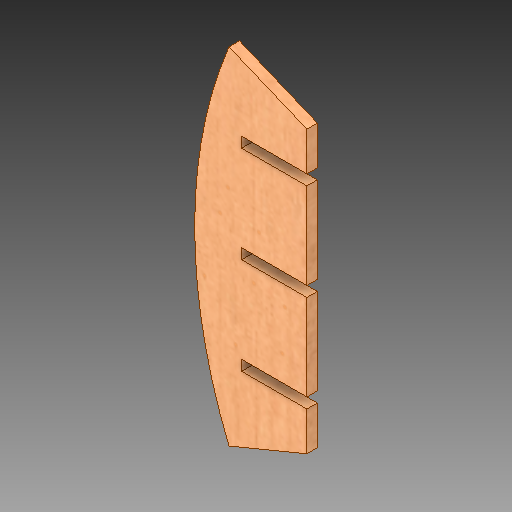
# Autodesk Inventor part: frontformer
Saved by Autodesk Inventor 2019 (Build 230136000, 136)
## iProperties
Company: FABLAB Torino
Created: 2019-01-11
Part Number: frontformer
Material: Wood (Cherry)
Document SubType Name: Modeling
Designer: Giancarlo
Density: 0.63 g/cm^3
Appearance: Cherry - Natural Low Gloss
Description: MultiLayer 4mm
Project: La Panca - Flower Vase
Author: Giancarlo
Title: La Panca - Flower Vase
Subject: Construction MOld
Autodesk Inventor part; units mm, degrees
ref_plane "YZ Plane" through (0, 0, 0) normal (1, 0, 0) x (0, 1, 0)
ref_plane "XZ Plane" through (0, 0, 0) normal (0, 1, 0) x (-1, 0, 0)
ref_plane "Work Plane1" through (0, 0, 0) normal (0, 0, 1) x (1, 0, 0)
sketch "Sketch1" plane through (0, 0, 0) normal (0, 0, 1) x (1, 0, 0)
  line L0 (300, 300) -> (-300, 300) construction
  line L1 (-300, 300) -> (-300, -300) construction
  line L2 (-300, -300) -> (300, -300) construction
  line L3 (300, -300) -> (300, 300) construction
  line L4 (300, -53.8478) -> (-254.3277, -283.4578) construction
  arc A0 (269.6349, -64.9002) -> (269.6349, -64.9002) centre (430, 0) ccw construction
  arc A1 (269.2287, 63.8872) -> (269.6349, -64.9002) centre (430, 0) ccw construction
  arc A2 (269.2287, 63.8872) -> (269.2287, 63.8872) centre (430, 0) ccw construction
  line L5 (-254.3277, 283.4578) -> (300, 53.8478) construction
  line L6 (300, 53.8478) -> (300, -53.8478)
  line L7 (270.1688, -66.2042) -> (300, -53.8478)
  line L8 (270.1688, 66.2042) -> (300, 53.8478)
  arc A3 (270.1688, 66.2042) -> (270.1688, -66.2042) centre (430, 0) ccw
  line L9 (300, -35) -> (275, -35)
  line L10 (275, -35) -> (275, -39)
  line L11 (275, -39) -> (300, -39)
  line L12 (300, -39) -> (300, -35)
  line L13 (300, 2) -> (275, 2)
  line L14 (275, 2) -> (275, -2)
  line L15 (275, -2) -> (300, -2)
  line L16 (300, -2) -> (300, 2)
  line L17 (300, 39) -> (275, 39)
  line L18 (275, 39) -> (275, 35)
  line L19 (275, 35) -> (300, 35)
  line L20 (300, 35) -> (300, 39)
  point P0 (0, 0)
  point P1 (300, 0)
  dimension "d2" = 25
  dimension "d3" = 4
  dimension "d4" = 25
  dimension "d5" = 4
  dimension "d6" = 25
  dimension "d7" = 4
  dimension "d8" = 35
  dimension "d9" = 35
  constraints: 30 end point, 6 parallel, 5 point on line, 3 horizontal, 3 perpendicular, 3 point on circle, 2 collinear, 2 midpoint, 1 centre point, 1 coincident
  measures "d2" distance of L11.end L10.end
  measures "d3" distance of L10.end L9.end
  measures "d4" distance of L15.end L14.end
  measures "d5" distance of L14.end L13.end
  measures "d6" distance of L19.end L18.end
  measures "d7" distance of L18.end L17.end
  measures "d8" distance from line of point (300, 0) L9
  measures "d9" distance from line of L19 point (300, 0)
extrude "Extrusion2" add sketch "Sketch1" along normal blind 4 contours L6 L17 L18 L19 L13 L14 L15 L9 L10 L11 L7 A3 L8
equation "\"d3\" = d7"
equation "\"d5\" = d7"
body "Solid2"
